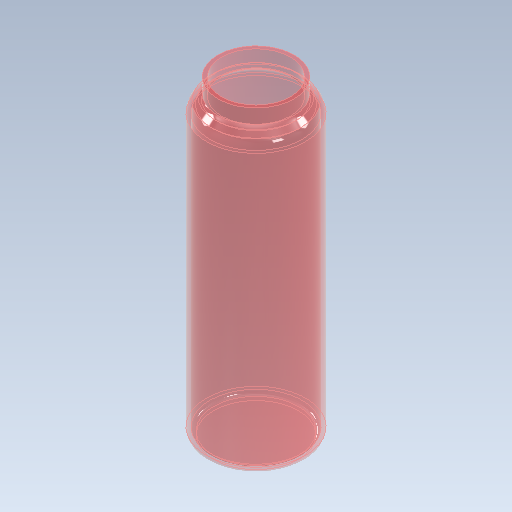
# Autodesk Inventor part: 40ml Bottle 1
Saved by Autodesk Inventor 2021 (Build 250183000, 183)
## iProperties
Created: 2019-11-05
Part Number: 40ml Bottle 1
Material: Glass
Document SubType Name: Modeling
Designer: jgray
Density: 2.18 g/cm^3
Appearance: Dark Red
Author: jgray
Autodesk Inventor part; units mm, degrees
ref_plane "YZ Plane" through (0, 0, 0) normal (1, 0, 0) x (0, 1, 0)
ref_plane "XZ Plane" through (0, 0, 0) normal (0, 1, 0) x (-1, 0, 0)
ref_plane "XY Plane" through (0, 0, 0) normal (0, 0, 1) x (1, 0, 0)
sketch "Sketch1" plane through (0, 0, 0) normal (0, 1, 0) x (-1, 0, 0)
  circle A0 centre (0, 0) radius 13.75
  dimension "d0" = 27.5
  constraints: 1 centre point, 1 coincident
  measures "d0" diameter of A0
extrude "Extrusion1" add sketch "Sketch1" along normal blind 82
sketch "Sketch2" plane through (0, 82, 0) normal (0, 1, 0) x (1, 0, 0)
  circle A0 centre (0, 0) radius 10.55
  dimension "d3" = 21.1
  constraints: 1 centre point, 1 coincident
  measures "d3" diameter of A0
extrude "Extrusion2" add sketch "Sketch2" along normal blind 4
chamfer "Chamfer1" distance 3 angle 45 1 edges at (13.75, 82, 0)
fillet "Fillet1" radius 4 2 edges at (10.75, 82, 0) (13.75, 79, 0)
fillet "Fillet2" radius 2 1 edges at (13.75, 0, 0)
shell "Shell1" thickness 1 removed faces 1 at (-2.6323, 86, 2.332)
body "Solid1"
